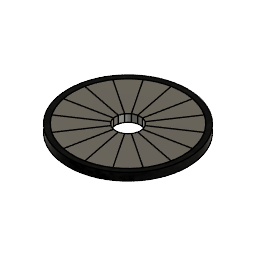
seal_land_assy (Autodesk Fusion 360 design; units mm, degrees)
part number: 2026-05-30-09-00-45-848
Autodesk Fusion 360 part; units mm, degrees
ref_plane "WorkPlane1" through (0, 0, 50.165) normal (0, 0, 1) x (1, 0, 0)
sketch "Sketch1" plane through (0, 0, 50.165) normal (0, 0, 1) x (1, 0, 0)
  arc A0 (22.2962, -4.435) -> (22.2962, 4.435) centre (0, 0) ccw
  line L0 (22.2962, 4.435) -> (99.9218, 19.8757)
  arc A1 (99.9218, -19.8757) -> (99.9218, 19.8757) centre (0, 0) ccw
  line L1 (99.9218, -19.8757) -> (22.2962, -4.435)
extrude "Extrude1" add sketch "Sketch1" along normal blind 13.97 makes body 1
ref_plane "WorkPlane2" through (0, 0, 50.165) normal (0, 0, 1) x (1, 0, 0)
sketch "Sketch2" plane through (0, 0, 50.165) normal (0, 0, 1) x (1, 0, 0)
  arc A0 (22.2962, 4.435) -> (18.9018, 12.6298) centre (0, 0) ccw
  line L0 (18.9018, 12.6298) -> (84.7096, 56.6012)
  arc A1 (99.9218, 19.8757) -> (84.7096, 56.6012) centre (0, 0) ccw
  line L1 (99.9218, 19.8757) -> (22.2962, 4.435)
extrude "Extrude2" add sketch "Sketch2" along normal blind 13.97 separate body makes body 2
ref_plane "WorkPlane3" through (0, 0, 50.165) normal (0, 0, 1) x (1, 0, 0)
sketch "Sketch3" plane through (0, 0, 50.165) normal (0, 0, 1) x (1, 0, 0)
  arc A0 (18.9018, 12.6298) -> (12.6298, 18.9018) centre (0, 0) ccw
  line L0 (12.6298, 18.9018) -> (56.6012, 84.7096)
  arc A1 (84.7096, 56.6012) -> (56.6012, 84.7096) centre (0, 0) ccw
  line L1 (84.7096, 56.6012) -> (18.9018, 12.6298)
extrude "Extrude3" add sketch "Sketch3" along normal blind 13.97 separate body makes body 3
ref_plane "WorkPlane4" through (0, 0, 50.165) normal (0, 0, 1) x (1, 0, 0)
sketch "Sketch4" plane through (0, 0, 50.165) normal (0, 0, 1) x (1, 0, 0)
  arc A0 (12.6298, 18.9018) -> (4.435, 22.2962) centre (0, 0) ccw
  line L0 (4.435, 22.2962) -> (19.8757, 99.9218)
  arc A1 (56.6012, 84.7096) -> (19.8757, 99.9218) centre (0, 0) ccw
  line L1 (56.6012, 84.7096) -> (12.6298, 18.9018)
extrude "Extrude4" add sketch "Sketch4" along normal blind 13.97 separate body makes body 4
ref_plane "WorkPlane5" through (0, 0, 50.165) normal (0, 0, 1) x (1, 0, 0)
sketch "Sketch5" plane through (0, 0, 50.165) normal (0, 0, 1) x (1, 0, 0)
  arc A0 (4.435, 22.2962) -> (-4.435, 22.2962) centre (0, 0) ccw
  line L0 (-4.435, 22.2962) -> (-19.8757, 99.9218)
  arc A1 (19.8757, 99.9218) -> (-19.8757, 99.9218) centre (0, 0) ccw
  line L1 (19.8757, 99.9218) -> (4.435, 22.2962)
extrude "Extrude5" add sketch "Sketch5" along normal blind 13.97 separate body makes body 5
ref_plane "WorkPlane6" through (0, 0, 50.165) normal (0, 0, 1) x (1, 0, 0)
sketch "Sketch6" plane through (0, 0, 50.165) normal (0, 0, 1) x (1, 0, 0)
  arc A0 (-4.435, 22.2962) -> (-12.6298, 18.9018) centre (0, 0) ccw
  line L0 (-12.6298, 18.9018) -> (-56.6012, 84.7096)
  arc A1 (-19.8757, 99.9218) -> (-56.6012, 84.7096) centre (0, 0) ccw
  line L1 (-19.8757, 99.9218) -> (-4.435, 22.2962)
extrude "Extrude6" add sketch "Sketch6" along normal blind 13.97 separate body makes body 6
ref_plane "WorkPlane7" through (0, 0, 50.165) normal (0, 0, 1) x (1, 0, 0)
sketch "Sketch7" plane through (0, 0, 50.165) normal (0, 0, 1) x (1, 0, 0)
  arc A0 (-12.6298, 18.9018) -> (-18.9018, 12.6298) centre (0, 0) ccw
  line L0 (-18.9018, 12.6298) -> (-84.7096, 56.6012)
  arc A1 (-56.6012, 84.7096) -> (-84.7096, 56.6012) centre (0, 0) ccw
  line L1 (-56.6012, 84.7096) -> (-12.6298, 18.9018)
extrude "Extrude7" add sketch "Sketch7" along normal blind 13.97 separate body makes body 7
ref_plane "WorkPlane8" through (0, 0, 50.165) normal (0, 0, 1) x (1, 0, 0)
sketch "Sketch8" plane through (0, 0, 50.165) normal (0, 0, 1) x (1, 0, 0)
  arc A0 (-18.9018, 12.6298) -> (-22.2962, 4.435) centre (0, 0) ccw
  line L0 (-22.2962, 4.435) -> (-99.9218, 19.8757)
  arc A1 (-84.7096, 56.6012) -> (-99.9218, 19.8757) centre (0, 0) ccw
  line L1 (-84.7096, 56.6012) -> (-18.9018, 12.6298)
extrude "Extrude8" add sketch "Sketch8" along normal blind 13.97 separate body makes body 8
ref_plane "WorkPlane9" through (0, 0, 50.165) normal (0, 0, 1) x (1, 0, 0)
sketch "Sketch9" plane through (0, 0, 50.165) normal (0, 0, 1) x (1, 0, 0)
  arc A0 (-22.2962, 4.435) -> (-22.2962, -4.435) centre (0, 0) ccw
  line L0 (-22.2962, -4.435) -> (-99.9218, -19.8757)
  arc A1 (-99.9218, 19.8757) -> (-99.9218, -19.8757) centre (0, 0) ccw
  line L1 (-99.9218, 19.8757) -> (-22.2962, 4.435)
extrude "Extrude9" add sketch "Sketch9" along normal blind 13.97 separate body makes body 9
ref_plane "WorkPlane10" through (0, 0, 50.165) normal (0, 0, 1) x (1, 0, 0)
sketch "Sketch10" plane through (0, 0, 50.165) normal (0, 0, 1) x (1, 0, 0)
  arc A0 (-22.2962, -4.435) -> (-18.9018, -12.6298) centre (0, 0) ccw
  line L0 (-18.9018, -12.6298) -> (-84.7096, -56.6012)
  arc A1 (-99.9218, -19.8757) -> (-84.7096, -56.6012) centre (0, 0) ccw
  line L1 (-99.9218, -19.8757) -> (-22.2962, -4.435)
extrude "Extrude10" add sketch "Sketch10" along normal blind 13.97 separate body makes body 10
ref_plane "WorkPlane11" through (0, 0, 50.165) normal (0, 0, 1) x (1, 0, 0)
sketch "Sketch11" plane through (0, 0, 50.165) normal (0, 0, 1) x (1, 0, 0)
  arc A0 (-18.9018, -12.6298) -> (-12.6298, -18.9018) centre (0, 0) ccw
  line L0 (-12.6298, -18.9018) -> (-56.6012, -84.7096)
  arc A1 (-84.7096, -56.6012) -> (-56.6012, -84.7096) centre (0, 0) ccw
  line L1 (-84.7096, -56.6012) -> (-18.9018, -12.6298)
extrude "Extrude11" add sketch "Sketch11" along normal blind 13.97 separate body makes body 11
ref_plane "WorkPlane12" through (0, 0, 50.165) normal (0, 0, 1) x (1, 0, 0)
sketch "Sketch12" plane through (0, 0, 50.165) normal (0, 0, 1) x (1, 0, 0)
  arc A0 (-12.6298, -18.9018) -> (-4.435, -22.2962) centre (0, 0) ccw
  line L0 (-4.435, -22.2962) -> (-19.8757, -99.9218)
  arc A1 (-56.6012, -84.7096) -> (-19.8757, -99.9218) centre (0, 0) ccw
  line L1 (-56.6012, -84.7096) -> (-12.6298, -18.9018)
extrude "Extrude12" add sketch "Sketch12" along normal blind 13.97 separate body makes body 12
ref_plane "WorkPlane13" through (0, 0, 50.165) normal (0, 0, 1) x (1, 0, 0)
sketch "Sketch13" plane through (0, 0, 50.165) normal (0, 0, 1) x (1, 0, 0)
  arc A0 (-4.435, -22.2962) -> (4.435, -22.2962) centre (0, 0) ccw
  line L0 (4.435, -22.2962) -> (19.8757, -99.9218)
  arc A1 (-19.8757, -99.9218) -> (19.8757, -99.9218) centre (0, 0) ccw
  line L1 (-19.8757, -99.9218) -> (-4.435, -22.2962)
extrude "Extrude13" add sketch "Sketch13" along normal blind 13.97 separate body makes body 13
ref_plane "WorkPlane14" through (0, 0, 50.165) normal (0, 0, 1) x (1, 0, 0)
sketch "Sketch14" plane through (0, 0, 50.165) normal (0, 0, 1) x (1, 0, 0)
  arc A0 (4.435, -22.2962) -> (12.6298, -18.9018) centre (0, 0) ccw
  line L0 (12.6298, -18.9018) -> (56.6012, -84.7096)
  arc A1 (19.8757, -99.9218) -> (56.6012, -84.7096) centre (0, 0) ccw
  line L1 (19.8757, -99.9218) -> (4.435, -22.2962)
extrude "Extrude14" add sketch "Sketch14" along normal blind 13.97 separate body makes body 14
ref_plane "WorkPlane15" through (0, 0, 50.165) normal (0, 0, 1) x (1, 0, 0)
sketch "Sketch15" plane through (0, 0, 50.165) normal (0, 0, 1) x (1, 0, 0)
  arc A0 (12.6298, -18.9018) -> (18.9018, -12.6298) centre (0, 0) ccw
  line L0 (18.9018, -12.6298) -> (84.7096, -56.6012)
  arc A1 (56.6012, -84.7096) -> (84.7096, -56.6012) centre (0, 0) ccw
  line L1 (56.6012, -84.7096) -> (12.6298, -18.9018)
extrude "Extrude15" add sketch "Sketch15" along normal blind 13.97 separate body makes body 15
ref_plane "WorkPlane16" through (0, 0, 50.165) normal (0, 0, 1) x (1, 0, 0)
sketch "Sketch16" plane through (0, 0, 50.165) normal (0, 0, 1) x (1, 0, 0)
  arc A0 (18.9018, -12.6298) -> (22.2962, -4.435) centre (0, 0) ccw
  line L0 (22.2962, -4.435) -> (99.9218, -19.8757)
  arc A1 (84.7096, -56.6012) -> (99.9218, -19.8757) centre (0, 0) ccw
  line L1 (84.7096, -56.6012) -> (18.9018, -12.6298)
extrude "Extrude16" add sketch "Sketch16" along normal blind 13.97 separate body makes body 16
ref_plane "WorkPlane17" through (0, 0, 50.165) normal (0, 0, 1) x (1, 0, 0)
sketch "Sketch17" plane through (0, 0, 50.165) normal (0, 0, 1) x (1, 0, 0)
  circle A0 centre (0, 0) radius 110.744
  circle A1 centre (0, 0) radius 101.8794
extrude "Extrude17" add sketch "Sketch17" along normal blind 13.97 separate body makes body 17
named bodies: "SHEX-005_petal_01", "SHEX-005_petal_02", "SHEX-005_petal_03", "SHEX-005_petal_04", "SHEX-005_petal_05", "SHEX-005_petal_06", "SHEX-005_petal_07", "SHEX-005_petal_08", "SHEX-005_petal_09", "SHEX-005_petal_10", "SHEX-005_petal_11", "SHEX-005_petal_12", "SHEX-005_petal_13", "SHEX-005_petal_14", "SHEX-005_petal_15", "SHEX-005_petal_16", "SHEX-004_cup_viz"
